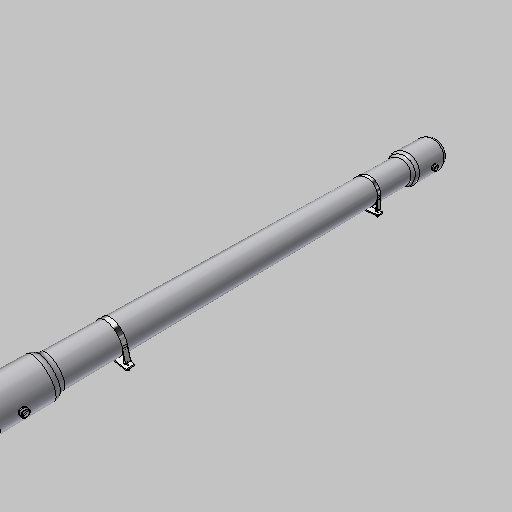
# Autodesk Inventor part: RO_PROTEC_ARISWA
Saved by Autodesk Inventor 2025.2 (Build 292293000, 293)
## iProperties
RuleStatus: InUse
Created: 2016-08-19
Part Number: RO_PROTEC_ARISWA
Material: CFRP
Document SubType Name: Modeling
Designer: Marc Crauwels
Density: 1.43 g/cm^3
Appearance: Chrome - Polished
Mass: 53965.4 g
Surface Area: 50032 cm^2
Volume: 37738 cm^3
AfterAnyParamChange0: Weight
Author: Marc Crauwels
Autodesk Inventor part; units mm, degrees
ref_plane "XY Plane" through (0, 0, 0) normal (0, 0, 1) x (1, 0, 0)
ref_plane "Work Plane4" through (0, 0, 0) normal (0, 0, -1) x (0, 1, 0)
sketch "Sketch3" plane through (0, 0, 0) normal (0, 0, -1) x (0, 1, 0)
  line L0 (0, -103) -> (0, 103) construction
  line L1 (-1766, 103) -> (1766, 103)
  line L2 (1766, 103) -> (1766, 108.5)
  line L3 (1766, 108.5) -> (-1766, 108.5)
  line L4 (-1766, 108.5) -> (-1766, 103)
  line L5 (-1766, 0) -> (1766, 0)
  line L6 (-1766, 108.5) -> (-1752.043, 120.25)
  arc A0 (-1719.8415, 132) -> (-1752.043, 120.25) centre (-1719.8415, 82) ccw
  line L7 (-1719.8415, 132) -> (-1430.403, 132)
  arc A1 (-1398.2015, 120.25) -> (-1430.403, 132) centre (-1430.403, 82) ccw
  arc A2 (-1398.2015, 120.25) -> (-1366, 108.5) centre (-1366, 158.5) ccw
  line L8 (-1398.2015, 120.25) -> (-1752.043, 120.25) construction
  line L9 (-1710, 103) -> (1710, 103)
  line L10 (1710, 103) -> (1710, 0)
  line L11 (1710, 0) -> (-1710, 0)
  line L12 (-1710, 0) -> (-1710, 103)
  line L13 (-1816.5, 87.15) -> (-1816.5, 83.47)
  line L14 (-1816.5, 83.47) -> (-1710, 83.47)
  line L15 (-1710, 83.47) -> (-1710, 87.15)
  line L16 (-1710, 63) -> (-1816.5, 63)
  line L17 (-1800.62, 87.15) -> (-1800.62, 85.545)
  line L18 (-1800.62, 85.545) -> (-1792.67, 85.545)
  line L19 (-1792.67, 85.545) -> (-1792.67, 87.15)
  line L20 (-1710, 87.15) -> (-1792.67, 87.15)
  line L21 (-1800.62, 87.15) -> (-1816.5, 87.15)
  line L22 (1710, 408.47) -> (1710, 412.15)
  line L23 (-1600.5, 108.5) -> (-1600.5, 152)
  line L24 (-1580.03, 108.5) -> (-1580.03, 152)
  line L25 (-1580.03, 152) -> (-1576.35, 152)
  line L26 (-1576.35, 152) -> (-1576.35, 136.12)
  line L27 (-1576.35, 136.12) -> (-1577.955, 136.12)
  line L28 (-1577.955, 136.12) -> (-1577.955, 128.17)
  line L29 (-1577.955, 128.17) -> (-1576.35, 128.17)
  line L30 (-1576.35, 128.17) -> (-1576.35, 108.5)
  line L31 (-1580.03, 108.5) -> (-1576.35, 108.5)
  line L32 (-1710, 16.85) -> (-1752.5, 16.85)
  line L33 (-1752.5, 16.85) -> (-1752.5, 20.85)
  line L34 (-1752.5, 20.85) -> (-1710, 20.85)
  line L35 (-1710, 20.85) -> (-1710, 16.85)
  line L36 (-1710, 12.85) -> (-1752.5, 12.85)
  line L37 (-1752.5, 12.85) -> (-1752.5, 16.85)
  line L38 (-1752.5, 16.85) -> (-1710, 16.85)
  line L39 (-1710, 16.85) -> (-1710, 12.85)
  line L40 (-1752.5, 15.85) -> (-1727.5, 15.85)
  line L41 (-1727.5, 15.85) -> (-1727.5, 12.85)
  line L42 (-1727.5, 12.85) -> (-1752.5, 12.85)
  line L43 (-1752.5, 12.85) -> (-1752.5, 15.85)
  line L44 (-1752.5, 15.85) -> (-1727.5, 15.85)
  line L45 (-1727.5, 15.85) -> (-1727.5, 20.85)
  line L46 (-1727.5, 20.85) -> (-1752.5, 20.85)
  line L47 (-1752.5, 20.85) -> (-1752.5, 15.85)
  line L48 (-1366, 108.5) -> (-1766, 108.5)
  point P0 (0, 0)
  point P1 (0, 0)
  point P2 (0, 0)
  point P3 (0, 0)
  dimension "d14" = 3532
  dimension "d15" = 217
  dimension "d16" = 50
  dimension "d17" = 400
  dimension "d18" = 264
  dimension "d19" = 56
  dimension "d20" = 63
  dimension "d23" = 106.5
  dimension "d24" = 15.88
  dimension "d25" = 7.95
  dimension "d26" = 45.09
  dimension "d27" = 48.3
  dimension "d28" = 3.68
  dimension "d33" = 48.3
  dimension "d34" = 152
  dimension "d35" = 33.7
  dimension "d36" = 25
  dimension "d38" = 4
  dimension "d39" = 64
  dimension "d40" = 1
  dimension "d41" = 152
  dimension "d105" = 206
  constraints: 98 end point, 21 point on line, 20 perpendicular, 17 parallel, 10 horizontal, 6 point on circle, 5 equal length, 5 tangent, 4 collinear, 4 midpoint, 3 centre point, 3 coincident, 2 equal radius, 1 vertical
  measures "d14" distance of L2.end L3.end
  measures "d15" diameter of L3 L5
  measures "d16" radius of A0
  measures "d17" distance of L48.start L3.end
  measures "d18" diameter of L7 L5
  measures "d19" distance between parallel lines of L12 L4
  measures "d20" distance between parallel lines of L16 L5
  measures "d23" distance of L15.end L13.start
  measures "d24" distance between parallel lines of L17 L13
  measures "d25" distance of L17.end L18.end
  measures "d26" diameter of L18 L16
  measures "d27" diameter of L20 L16
  measures "d28" distance between parallel lines of L14 L20
  measures "d33" diameter of L26 L23
  measures "d34" vertical distance of L23.end L11.end
  measures "d35" diameter of L32 L5
  measures "d36" distance of L40.end L44.start
  measures "d38" distance of L36.end L32.end
  measures "d39" distance between parallel lines of L13 L47
  measures "d40" distance between parallel lines of L40 L38
  measures "d41" distance from line of L33 L23.end
  measures "d105" diameter of L9 L5
revolve "Corps" add sketch "Sketch3" angle 360 about axis through (0, -1766, 0) along (0, 1, 0) contours L4 L3 L2 L1
revolve "BellPermeateSide" add sketch "Sketch3" angle 360 about axis through (0, 1710, 0) along (0, -1, 0) contours L6 A0 L7 L23 L3 | L23 L7 L24 L3 | L24 L7 L28 L29 L30 L3 | L30 L29 L28 L7 A1 A2 L3
mirror "BellBackSide" about plane through (0, 0, 0) normal (0, 1, 0) of "BellPermeateSide"
revolve "Inside" add sketch "Sketch3" angle 360 about axis through (0, 1710, 0) along (0, -1, 0) contours L1 L10 L5 L12
revolve "ConcentrateSideNozzle" add sketch "Sketch3" angle 360 about axis through (108.5, -1600.5, 0) along (1, 0, 0) separate body contours L24 L7 L28 L29 L30 L3 | L24 L25 L26 L27 L28 L7
pattern_linear "FeedSideNozzle" count 2 spacing 3200 along (0, 1, 0) bodies 2
revolve "ConcentrateEndNozzle" [suppressed]
mirror "FeedEndNozzle" [suppressed]
revolve "PermeateNozzle" add sketch "Sketch3" angle 360 about axis through (0, -1766, 0) along (0, 1, 0) separate body contours L36 L41 L45 L32 L12 | L12 L32 L45 L34 | L36 L37 L40 L41 | L45 L32 L33 L34 | L45 L40 L37 L32
revolve "MaleTRD" [suppressed]
revolve "FemaleTRD" cut sketch "Sketch3" angle 360 about axis through (0, -1766, 0) along (0, 1, 0) bodies 3 contours L36 L37 L40 L41
mirror "Mirror3" about plane through (0, 0, 0) normal (0, 1, 0) bodies 3
ref_plane "Work Plane2" through (0, -1016, 0) normal (0, 1, 0) x (-1, 0, 0)
sketch "Sketch6" plane through (0, -1016, 0) normal (0, 1, 0) x (-1, 0, 0)
  circle A0 centre (0, 0) radius 108.5
  circle A1 centre (0, 0) radius 110.5
  line L0 (-109.8458, 12.0063) -> (-121.4586, -94.2394)
  arc A2 (-120.4645, -94.3481) -> (-108.5003, -94.9364) centre (-114.5, -95) ccw
  arc A3 (-121.4586, -94.2394) -> (-107.5004, -94.9258) centre (-114.5, -95) ccw
  line L1 (-107.5004, -94.9258) -> (-108.4939, -1.1494)
  circle A4 centre (0, 0) radius 109.5
  line L2 (-108.8517, 11.8976) -> (-120.4645, -94.3481)
  line L3 (0, 0) -> (0, -125)
  line L4 (114.5, -125) -> (-114.5, -125)
  line L5 (-114.5, -125) -> (-114.5, -95) construction
  line L6 (-108.5003, -94.9364) -> (-109.4939, -1.16)
  line L7 (135, -125) -> (-135, -125)
  line L8 (-135, -125) -> (-135, -115)
  line L9 (-135, -115) -> (135, -115)
  line L10 (135, -115) -> (135, -125)
  line L11 (75, -81.1496) -> (-75, -81.1496)
  line L12 (-75, -81.1496) -> (-75, -115)
  line L13 (-75, -115) -> (75, -115)
  line L14 (75, -115) -> (75, -81.1496)
  line L15 (-108.8517, 11.8976) -> (-109.8458, 12.0063)
  line L16 (-109.4939, -1.16) -> (-108.4939, -1.1494)
  circle A5 centre (-114.5, -95) radius 6
  point P0 (0, 0)
  point P1 (-108.5, 0)
  point P2 (-108.5, 0)
  point P3 (-108.5, 0)
  point P4 (0, 0)
  point P5 (0, 0)
  point P6 (0, 0)
  dimension "d62" = 2
  dimension "d63" = 6
  dimension "d64" = 1
  dimension "d65" = 125
  dimension "d66" = 229
  dimension "d67" = 30
  dimension "d69" = 270
  dimension "d70" = 10
  dimension "d71" = 150
  constraints: 34 end point, 11 point on circle, 8 tangent, 5 centre point, 5 parallel, 3 coincident, 3 horizontal, 3 perpendicular, 2 midpoint, 2 vertical, 1 concentric, 1 point on line, 3 other
  measures "d62" radial gap between concentric circles of A0 A1
  measures "d63" radius of A2
  measures "d64" radial gap between concentric circles of A0 A4
  measures "d65" distance of L3.end L3.start
  measures "d66" distance of L4.start L4.end
  measures "d67" distance of L4.end L5.end
  measures "d69" distance of L8.end L9.end
  measures "d70" distance of L7.end L8.end
  measures "d71" distance of L11.start L11.end
extrude "Extrusion1" add sketch "Sketch6" along normal mid plane 32 separate body contours A0 L11 | A0 L16 A4 L11 | A0 L11 A4 L1 | L1 A4 L16 | L11 A4 L3 A0 | A0 L3 L11 | L11 L3 A0 | A0 L3 A4 L11 | A4 L11 A1 L1 | L1 A1 L6 A4 | L6 A1 L2 A4 | L11 A1 L3 A4 | A4 L15 A1 L11 | A4 L3 A1 L11 | L2 A1 L15
extrude "Extrusion2" add sketch "Sketch6" along normal mid plane 32 contours L1 A4 L16 | L1 A1 L6 A4 | L1 A3 L0 A1 L2 A2 L6 | L2 A1 L15 bodies 4
extrude "Extrusion4" add sketch "Sketch6" along normal mid plane 40 contours A2 A5 bodies 4
mirror "Mirror4" about plane through (0, 0, 0) normal (1, 0, 0) bodies 4
extrude "Extrusion3" add sketch "Sketch6" along normal mid plane 52 contours L9 L10 L7 L4 L3 | L9 L3 L4 L7 L8 bodies 4
sketch "Sketch7" plane through (135, -990, -125) normal (0, 0, -1) x (-1, 0, 0)
  point P0 (135, 990)
  point P1 (249.5, -26)
  point P2 (20.5, -26)
hole "Hole1" at (-114.5, -1016, -125) at (114.5, -1016, -125) direction (0, 0, 1) diameter 10 depth 30 tip angle 118 bodies 4
sketch "Sketch8" plane through (135, -990, -125) normal (0, 0, -1) x (-1, 0, 0)
  circle A0 centre (20.5, -26) radius 5 projected
  circle A1 centre (20.5, -26) radius 4
  point P0 (135, 990)
  dimension "d87" = 8
  constraints: 1 centre point, 1 coincident
  measures "d87" diameter of A1
extrude "Extrusion5" add sketch "Sketch8" along normal blind 15 contours A1 bodies 4
sketch "Sketch9" plane through (114.5, -1016, -140) normal (0, 0, -1) x (-1, 0, 0)
  circle A0 centre (0, 0) radius 4 projected
  line L0 (-3.7528, 6.5) -> (3.7528, 6.5)
  line L1 (3.7528, 6.5) -> (7.5056, 0)
  line L2 (7.5056, 0) -> (3.7528, -6.5)
  line L3 (3.7528, -6.5) -> (-3.7528, -6.5)
  line L4 (-3.7528, -6.5) -> (-7.5056, 0)
  line L5 (-7.5056, 0) -> (-3.7528, 6.5)
  point P0 (114.5, 1016)
  dimension "d90" = 13
  constraints: 12 end point, 1 coincident, 1 horizontal, 13 other
  measures "d90" distance between parallel lines of L5 L2
extrude "Extrusion6" add sketch "Sketch9" along normal blind 8 contours A0 | L0 L1 L2 L3 L4 L5 bodies 4
sketch "Sketch10" plane through (114.5, -1016, -125) normal (0, 0, 1) x (1, 0, 0)
  circle A0 centre (0, 0) radius 4 projected
  point P0 (-114.5, 1016)
extrude "Extrusion7" add sketch "Sketch10" along normal blind 35 bodies 4
mirror "Mirror5" about plane through (0, 0, 0) normal (1, 0, 0) of "Extrusion5", "Extrusion6", "Extrusion7" bodies 4
pattern_linear "Rectangular Pattern2" count 2 spacing 2032 along (0, 1, 0) bodies 4
sketch "Sketch13" plane through (0, 0, 0) normal (1, 0, 0) x (0, 1, 0)
  line L0 (-1510, 0) -> (1510, 0)
  line L1 (1510, 0) -> (1510, 101)
  line L2 (1510, 101) -> (-1510, 101)
  line L3 (-1510, 101) -> (-1510, 0)
  line L4 (-1710, -103) -> (-1710, 103) projected
  line L5 (-1366, 108.5) -> (1366, 108.5) projected
  point P0 (0, 0)
  point P1 (0, 0)
  dimension "d107" = 200
  dimension "d110" = 101
  constraints: 8 end point, 2 parallel, 1 coincident, 1 horizontal, 1 midpoint, 1 perpendicular
  measures "d107" distance between parallel lines of L4 L3
  measures "d110" distance between parallel lines of L2 L0
revolve "Revolution11" cut sketch "Sketch13" angle 360 about axis through (0, -1510, 0) along (0, 1, 0) bodies 1
equation "\"d14\" = ShellLenght"
equation "\"d15\" = VesselDiameter"
equation "\"d17\" = BellLenght"
equation "\"d18\" = MaximumBell"
equation "\"d19\" = BearingPlateOffset"
equation "\"d23\" = NozzleEFlenght"
equation "\"d33\" = d27"
equation "\"d34\" = SideNozzleOffset"
equation "\"d39\" = PermeateNozzleOffset"
equation "\"d41\" = SideNozzleDist"
equation "\"SideNozzels\" = 1"
equation "\"EndNozzles\" = 0"
equation "\"LenghtFilterElement\" = 1016"
equation "\"VesselDiameter\" = 217"
equation "\"MaximumBell\" = 264"
equation "\"BellLenght\" = 400"
equation "\"BearingPlateOffset\" = 56"
equation "\"NozzleEFlenght\" = 106.5"
equation "\"PermeateNozzleOffset\" = 64"
equation "\"SideNozzleDist\" = 152"
equation "\"BasicSideNozzleCenterCenter\" = 1168"
equation "\"SideNozzleOffset\" = 152"
equation "\"SupportDistance\" = 2032"
equation "\"ShellLenght\" = 3532"
body "Solid2"
body "Solid5"
body "Solid6"
body "Solid7"
body "Solid8"
body "Solid9"
body "Solid10"
body "Solid11"
